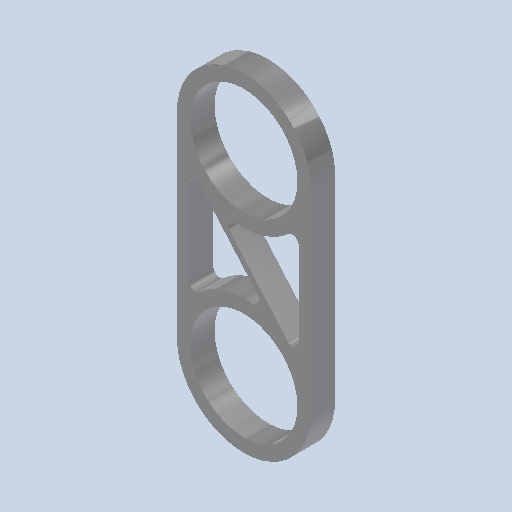
# Autodesk Inventor part: BRACE,SHAFT,ELEVATOR
Saved by Autodesk Inventor 2025.2 (Build 292293000, 293)
## iProperties
ILogicPurgeVersion: 0.0.0.0
OnSaveVersion: 3.5.0.0
OnSaveAssembly: COREAutomationManager
Category: _
Manager: _
Created: 2025-03-04
Part Number: BRACE,SHAFT,ELEVATOR
Checked By: 00
Engr Approved By: _
User Status: Work In Process
Material: Aluminum 7075
Description: STANDARD (mm)
Document SubType Name: Modeling
Mfg Approved By: John.Thibert
Designer: John.Thibert
Manufacturer: Standard
Standards Organization: Custom
Mass: 17.7363 g
Surface Area: 53.5584 cm^2
Volume: 6.31186 cm^3
Density: 2.81 g/cm^3
Appearance: Aluminum - Polished
CN_MASS: 0.02
CN_SERVICEABLE: _
FIRST_DESCRIPTION: _
SECOND_DESCRIPTION: _
THIRD_DESCRIPTION: _
ModelCat: Uncategorized
MaterialName: Aluminum 7075
Subject: _
Author: John.Thibert
Keywords: -
Revision Number: A
Autodesk Inventor part; units mm, degrees
ref_plane "YZ Plane" through (0, 0, 0) normal (1, 0, 0) x (0, 1, 0)
ref_plane "XZ Plane" through (0, 0, 0) normal (0, 1, 0) x (-1, 0, 0)
ref_plane "XY Plane" through (0, 0, 0) normal (0, 0, 1) x (1, 0, 0)
sketch "Sketch2" plane through (0, 0, 0) normal (0, 0, 1) x (1, 0, 0)
  line L0 (0, -25.4) -> (0, 25.4) construction
  line L1 (17.4625, -25.4) -> (17.4625, 25.4)
  line L2 (-17.4625, 25.4) -> (-17.4625, -25.4)
  circle A0 centre (0, -25.4) radius 14.2875 construction
  circle A1 centre (0, 25.4) radius 14.2875 construction
  line L3 (-14.2875, -15.3598) -> (-14.2875, 15.218)
  line L4 (7.2043, -9.4928) -> (-14.2875, 15.218)
  line L5 (14.2875, -15.218) -> (-7.2043, 9.4928)
  line L6 (14.2875, -15.218) -> (14.2875, 15.3598)
  arc A2 (-17.4625, -25.4) -> (17.4625, -25.4) centre (0, -25.4) ccw
  arc A3 (7.2043, -9.4928) -> (-14.2875, -15.3598) centre (0, -25.4) ccw
  arc A4 (17.4625, 25.4) -> (-17.4625, 25.4) centre (0, 25.4) ccw
  arc A5 (-7.2043, 9.4928) -> (14.2875, 15.3598) centre (0, 25.4) ccw
  point P0 (0, 0)
  dimension "d3" = 28.575
  dimension "d4" = 50.8
  dimension "d15" = 1.5875
  dimension "d16" = 17.4625
  dimension "d18" = 3.175
  constraints: 16 end point, 8 point on circle, 6 centre point, 6 tangent, 4 parallel, 3 equal radius, 2 coincident, 2 vertical, 1 midpoint
  measures "d3" diameter of A0
  measures "d4" distance of L0.start L0.end
  measures "d15" distance between parallel lines of L5 L4
  measures "d16" radius of A2
  measures "d18" distance between parallel lines of L2 L3
extrude "Extrusion1" add sketch "Sketch2" along normal mid plane 6.35
sketch "Sketch3" plane through (0, 0, 3.175) normal (0, 0, 1) x (1, 0, 0)
  arc A0 (-17.4625, -25.4) -> (17.4625, -25.4) centre (0, -25.4) ccw construction
  arc A1 (17.4625, 25.4) -> (-17.4625, 25.4) centre (0, 25.4) ccw construction
  point P0 (0, 0)
  point P1 (0, 25.4)
  constraints: 2 coincident
hole "Hole1" at (0, -25.4, 3.175) at (0, 25.4, 3.175) direction (0, 0, -1) diameter 27.94 end through all
fillet "Fillet1" radius 1.5875 6 edges at (14.2875, -15.218, 0) (7.2043, -9.4928, 0) (14.2875, 15.3598, 0) (-7.2043, 9.4928, 0) (-14.2875, -15.3598, 0) (-14.2875, 15.218, 0)
body "Solid1"
